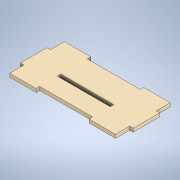
# Autodesk Inventor part: Platte3-Seite
Saved by Autodesk Inventor 2020.3 (Build 243373000, 373)
## iProperties
Created: 2020-11-28
Part Number: Platte3-Seite
Material: Generisch
Document SubType Name: Modeling
Designer: Stefan
Density: 1 g/cm^3
Appearance: Pappel
Author: Stefan
Autodesk Inventor part; units mm, degrees
ref_plane "YZ Plane" through (0, 0, 0) normal (1, 0, 0) x (0, 1, 0)
ref_plane "XZ Plane" through (0, 0, 0) normal (0, 1, 0) x (-1, 0, 0)
ref_plane "XY Plane" through (0, 0, 0) normal (0, 0, 1) x (1, 0, 0)
sketch "Skizze1" plane through (0, 0, 0) normal (0, 1, 0) x (-1, 0, 0)
  line L0 (-101.4396, -103.5796) -> (-101.4396, -93.5796)
  line L1 (-101.4396, -93.5796) -> (48.5604, -93.5796)
  line L2 (48.5604, -93.5796) -> (48.5604, -103.5796)
  line L3 (-176.4396, -103.5796) -> (-101.4396, -103.5796)
  line L4 (48.5604, -103.5796) -> (123.5604, -103.5796)
  line L5 (-101.4396, 51.4204) -> (-101.4396, 41.4204)
  line L6 (-101.4396, 41.4204) -> (48.5604, 41.4204)
  line L7 (48.5604, 41.4204) -> (48.5604, 51.4204)
  line L8 (123.5604, 51.4204) -> (48.5604, 51.4204)
  line L9 (-101.4396, 51.4204) -> (-176.4396, 51.4204)
  line L10 (123.5604, 11.4204) -> (133.5604, 11.4204)
  line L11 (133.5604, 11.4204) -> (133.5604, -63.5796)
  line L12 (133.5604, -63.5796) -> (123.5604, -63.5796)
  line L13 (123.5604, -103.5796) -> (123.5604, -63.5796)
  line L14 (123.5604, 11.4204) -> (123.5604, 51.4204)
  line L15 (48.5604, -8.5796) -> (-101.4396, -8.5796)
  line L16 (-101.4396, -8.5796) -> (-101.4396, -18.5796)
  line L17 (-101.4396, -18.5796) -> (48.5604, -18.5796)
  line L18 (48.5604, -18.5796) -> (48.5604, -8.5796)
  line L19 (-176.4396, 11.4204) -> (-186.4396, 11.4204)
  line L20 (-186.4396, 11.4204) -> (-186.4396, -63.5796)
  line L21 (-186.4396, -63.5796) -> (-176.4396, -63.5796)
  line L22 (-176.4396, 51.4204) -> (-176.4396, 11.4204)
  line L23 (-176.4396, -63.5796) -> (-176.4396, -103.5796)
  dimension "d0" = 300
  dimension "d2" = 150
  dimension "d3" = 10
  dimension "d6" = 10
  dimension "d7" = 10
  dimension "d8" = 75
  dimension "d10" = 150
  dimension "d11" = 10
  dimension "d13" = 10
  dimension "d14" = 75
  dimension "d17" = 10
  dimension "d20" = 10
  dimension "d22" = 50
  dimension "d25" = 155
  dimension "d26" = 0
  dimension "d27" = 10
  dimension "d28" = 40
  dimension "d29" = 40
  dimension "d30" = 85
  dimension "d31" = 75
  dimension "d32" = 85
  dimension "d33" = 75
  dimension "d34" = 10
  dimension "d35" = 150
  constraints: 48 end point, 14 parallel, 7 perpendicular, 5 horizontal
  measures "d0" distance of L4.end L3.start
  measures "d2" distance of L0.end L1.end
  measures "d3" distance of L0.start L0.end
  measures "d6" distance of L5.end L5.start
  measures "d7" distance of L11.end L12.end
  measures "d8" distance of L10.end L11.end
  measures "d10" distance of L17.end L16.end
  measures "d11" distance of L16.end L15.end
  measures "d13" distance of L21.end L20.end
  measures "d14" distance of L20.end L19.end
  measures "d17" distance between parallel lines of L8 L6
  measures "d20" distance of L1.end L2.end
  measures "d22" distance between parallel lines of L6 L15
  measures "d25" distance between parallel lines of L3 L9
  measures "d26" horizontal distance of L7.end L6.end
  measures "d27" distance of L10.start L10.end
  measures "d28" distance between parallel lines of L4 L12
  measures "d29" distance between parallel lines of L3 L21
  measures "d30" distance between parallel lines of L20 L16
  measures "d31" distance between parallel lines of L23 L0
  measures "d32" distance between parallel lines of L11 L18
  measures "d33" distance from line of L22 L5.start
  measures "d34" distance of L19.start L19.end
  measures "d35" distance of L5.end L6.end
extrude "Extrusion1" add sketch "Skizze1" along normal blind 10
